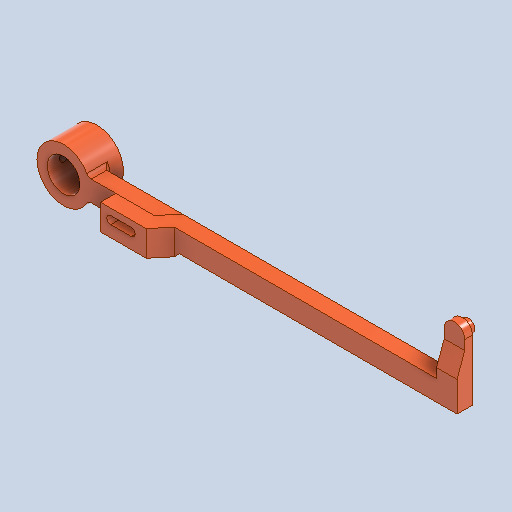
# Autodesk Inventor part: head_lock_2
Saved by Autodesk Inventor 2024 (Build 280153000, 153)
## iProperties
Created: 2021-06-14
Part Number: head_lock_2
Material: Generic
Document SubType Name: Modeling
Designer: dsdan
Density: 1 g/cm^3
Appearance: Smooth - Light Orange
Author: dsdan
Autodesk Inventor part; units mm, degrees
ref_plane "YZ Plane" through (0, 0, 0) normal (1, 0, 0) x (0, 1, 0)
sketch "Sketch1" plane through (0, 0, 0) normal (0, 0, 1) x (1, 0, 0)
  circle A0 centre (7.936401, -24.412437) radius 2.575 construction
  circle A1 centre (7.936401, -24.412437) radius 2.55
  dimension "d70" = 5.1
  constraints: 1 centre point, 1 coincident
  measures "d70" diameter of A1
sketch "Sketch1 outline for Extrusion1" plane through (0, 0, 0) normal (0, 0, 1) x (1, 0, 0)
  circle A0 centre (7.936401, -24.412437) radius 2.55
extrude "Extrusion1" add sketch "Sketch1 outline for Extrusion1" against normal blind 2.4
sketch "Sketch2" plane through (0, 0, 0) normal (0, 0, 1) x (1, 0, 0)
  arc A0 (11.936401, -24.412437) -> (3.936401, -24.412437) centre (7.936401, -24.412437) ccw
  line L0 (11.936401, -24.412437) -> (3.936401, -24.412437) construction
  line L1 (3.936401, -24.412437) -> (3.936401, -40.089664)
  line L2 (11.936401, -48.089664) -> (11.936401, -24.412437)
  line L3 (-141.474726, -48.126865) -> (-141.474726, -40.126865) construction
  line L4 (-131.928915, -40.089664) -> (3.936401, -40.089664)
  arc A1 (-131.928915, -40.089664) -> (-131.928915, -48.089664) centre (-141.474726, -44.089664) ccw
  line L5 (11.936401, -48.089664) -> (-131.928915, -48.089664)
  circle A2 centre (-141.474726, -44.089664) radius 6.35
  line L6 (-118.52781, -40.089664) -> (-118.52781, -48.089664) construction
  circle A3 centre (-141.474726, -44.089664) radius 5.8293
  circle A4 centre (7.936401, -24.412437) radius 2.55
  point P0 (-118.52781, -44.089664)
  point P1 (12.740451, -19.012437)
  dimension "d3" = 8
  dimension "d36" = 12.7
  dimension "d37" = 4
  dimension "d38" = 8
  constraints: 14 end point, 4 point on circle, 3 centre point, 3 coincident, 3 perpendicular, 3 point on line, 2 horizontal, 2 parallel, 2 tangent, 1 concentric, 1 horizontal alignment, 1 midpoint, 1 other
  measures "d3" diameter of A0
  measures "d36" diameter of A2
  measures "d37" radial gap between concentric circles of A1 A2
  measures "d38" distance between parallel lines of L5 L4
sketch "Sketch2 outline for Extrusion2" plane through (0, 0, 0) normal (0, 0, 1) x (1, 0, 0)
  line L0 (11.936401, -48.089664) -> (11.936401, -24.412437)
  line L1 (-131.928915, -48.089664) -> (11.936401, -48.089664)
  arc A0 (11.936401, -24.412437) -> (3.936401, -24.412437) centre (7.936401, -24.412437) ccw
  arc A1 (-131.928915, -40.089664) -> (-131.928915, -48.089664) centre (-141.474726, -44.089664) ccw
  line L2 (3.936401, -24.412437) -> (3.936401, -40.089664)
  line L3 (3.936401, -40.089664) -> (-131.928915, -40.089664)
  circle A2 centre (-141.474726, -44.089664) radius 6.35
extrude "Extrusion2" add sketch "Sketch2 outline for Extrusion2" along normal blind 6
sketch "Sketch3" plane through (3.936401, -40.089664, 0) normal (-1, 0, 0) x (0, 0, 1)
  line L0 (0, 19.677227) -> (6, 19.677227)
  line L1 (3, 19.677227) -> (3, 11.919659)
  line L2 (3, 11.919659) -> (6, 3.677227)
  line L3 (6, 15.677227) -> (6, 19.677227)
  line L4 (6, 15.677227) -> (6, 0)
  point P0 (0, 40.089664)
  point P1 (5, 8)
  dimension "d8" = 160
  dimension "d10" = 16
  constraints: 4 end point, 1 midpoint, 1 perpendicular, 2 other
  measures "d8" angle of L1 L2
  measures "d10" distance of L0.end L2.end
sketch "Sketch3 outline for Extrusion3" plane through (3.936401, -40.089664, 0) normal (-1, 0, 0) x (0, 0, 1)
  line L0 (6, 15.677227) -> (6, 19.677227)
  line L1 (6, 3.677227) -> (6, 15.677227)
  line L2 (3, 11.919659) -> (6, 3.677227)
  line L3 (3, 19.677227) -> (3, 11.919659)
  line L4 (6, 19.677227) -> (3, 19.677227)
extrude "Extrusion3" cut sketch "Sketch3 outline for Extrusion3" against normal through all
ref_plane "Work Plane3" through (-155.900182, -65.296024, -7) normal (0, 0, 1) x (1, 0, 0)
sketch "Sketch8" plane through (-124.033402, -23.677227, 0) normal (0, 0, 1) x (1, 0, 0)
  arc A0 (-7.895513, -16.412437) -> (-7.895513, -24.412437) centre (-17.441324, -20.412437) ccw
  circle A1 centre (-17.441324, -20.412437) radius 6.35
  circle A2 centre (-17.441324, -20.412437) radius 10.35
  point P0 (124.033402, 23.677227)
  point P1 (-7.895513, -24.412437)
  point P2 (-7.895513, -16.412437)
  constraints: 1 centre point, 1 coincident, 1 concentric
sketch "Sketch8 outline for Extrusion8" plane through (-124.033402, -23.677227, 0) normal (0, 0, 1) x (1, 0, 0)
  arc A0 (-7.895513, -24.412437) -> (-7.895513, -16.412437) centre (-17.441324, -20.412437) ccw
  arc A1 (-7.895513, -16.412437) -> (-7.895513, -24.412437) centre (-17.441324, -20.412437) ccw
  circle A2 centre (-17.441324, -20.412437) radius 6.35
extrude "Extrusion8" add sketch "Sketch8 outline for Extrusion8" against normal up to surface (7 mm away)
fillet "Fillet1" radius 2 3 edges at (-131.1247, -44.0897, 0) (-131.9289, -48.0897, 3) (-131.9289, -40.0897, 3)
ref_plane "Work Plane2" through (-151.824726, -44.089664, 0) normal (-1, 0, 0) x (0, 0, 1)
sketch "Sketch9" plane through (-151.824726, -44.089664, 0) normal (-1, 0, 0) x (0, 0, 1)
  circle A0 centre (-0.5, 0) radius 1.8
  line L0 (6, -10.35) -> (6, 10.35) projected
  point P0 (0, 44.089664)
  point P1 (6, 5.02834)
  point P2 (6, -5.02834)
  point P3 (6, 0)
  dimension "d31" = 3.6
  dimension "d41" = 6.5
  constraints: 1 centre point, 1 horizontal alignment, 1 midpoint
  measures "d31" diameter of A0
  measures "d41" distance from line of A0.centre L0
sketch "Sketch9 outline for Extrusion9" plane through (-151.824726, -44.089664, 0) normal (-1, 0, 0) x (0, 0, 1)
  circle A0 centre (-0.5, 0) radius 1.8
extrude "Extrusion9" cut sketch "Sketch9 outline for Extrusion9" against normal up to next
sketch "Sketch10" plane through (11.936401, -48.089664, 0) normal (0, -1, 0) x (1, 0, 0)
  line L0 (-8, 6) -> (-142.616568, 6)
  line L1 (-118, 6) -> (-113, 0)
  line L2 (-8, 0) -> (-141.726842, 0)
  point P0 (-11.936401, 0)
  point P1 (-142.616879, 0)
  point P2 (-143.760295, 0)
  constraints: 2 end point, 2 point on line
surface extrude "ExtrusionSrf1" sketch "Sketch10" against normal through all shown no curves L1
split body "Split1" result two bodies by surface "ExtrusionSrf1" first body at (-134.013926, -50.520758, -1)
sketch "Sketch11" plane through (11.936401, -48.089664, 0) normal (0, -1, 0) x (1, 0, 0)
  line L0 (-8, 6) -> (-118, 6)
  line L1 (-110.18975, 6) -> (-115.18975, 12)
  line L2 (-110.18975, 6) -> (-102.379501, 6) construction
  line L3 (-115.18975, 12) -> (-133, 12)
  line L4 (-133, 12) -> (-133, 6)
  line L5 (-142.616568, 6) -> (-118, 6)
  line L6 (-133, 6) -> (-118, 6)
  line L7 (-118, 6) -> (-113, 0)
  line L8 (-118, 6) -> (-110.18975, 6)
  line L9 (-113, 0) -> (-141.726842, 0)
  line L10 (-113, 0) -> (0, 0)
  point P0 (-11.936401, 0)
  point P1 (-142.616879, 0)
  point P2 (-143.760295, 0)
  dimension "d47" = 6
  dimension "d48" = 6
  dimension "d49" = 15
  dimension "d64" = 6
  constraints: 12 end point, 2 horizontal, 1 collinear, 1 equal length, 1 parallel, 1 perpendicular, 1 point on line
  measures "d47" vertical distance of L1.start L1.end
  measures "d48" distance between parallel lines of L7 L1
  measures "d49" distance from line of L0.end L4
  measures "d64" distance between parallel lines of L10 L0
sketch "Sketch11 outline for Extrusion10" plane through (11.936401, -48.089664, 0) normal (0, -1, 0) x (1, 0, 0)
  line L0 (-115.18975, 12) -> (-133, 12)
  line L1 (-110.18975, 6) -> (-115.18975, 12)
  line L2 (-118, 6) -> (-110.18975, 6)
  line L3 (-133, 6) -> (-118, 6)
  line L4 (-133, 12) -> (-133, 6)
extrude "Extrusion10" add sketch "Sketch11 outline for Extrusion10" against normal up to surface (8 mm away) bodies 3
sketch "Sketch12" plane through (-121.063599, -48.089664, 12) normal (0, 0, 1) x (1, 0, 0)
  line L0 (4, 4) -> (12, 4) construction
  line L1 (4, 2.45) -> (12, 2.45)
  line L2 (12, 5.55) -> (4, 5.55)
  arc A0 (4, 5.55) -> (4, 2.45) centre (4, 4) ccw
  arc A1 (12, 2.45) -> (12, 5.55) centre (12, 4) ccw
  line L3 (0, 0) -> (0, 8)
  line L4 (17.81025, 0) -> (17.81025, 8)
  point P0 (121.063599, 48.089664)
  point P1 (8, 4)
  point P2 (0, 4)
  dimension "d52" = 8
  dimension "d53" = 3.1
  dimension "d54" = 4
  constraints: 8 end point, 4 point on circle, 4 tangent, 2 centre point, 2 midpoint, 1 horizontal, 1 parallel, 1 point on line
  measures "d52" distance of L0.start L0.end
  measures "d53" diameter of A1
  measures "d54" distance from line of L3 L0.start
sketch "Sketch12 outline for Extrusion11" plane through (-121.063599, -48.089664, 12) normal (0, 0, 1) x (1, 0, 0)
  line L0 (4, 2.45) -> (12, 2.45)
  arc A0 (4, 5.55) -> (4, 2.45) centre (4, 4) ccw
  line L1 (12, 5.55) -> (4, 5.55)
  arc A1 (12, 2.45) -> (12, 5.55) centre (12, 4) ccw
extrude "Extrusion11" cut sketch "Sketch12 outline for Extrusion11" against normal through all bodies 3
sketch "Sketch13" plane through (0, 0, 6) normal (0, 0, 1) x (1, 0, 0)
  arc A0 (-109.063599, -45.639664) -> (-109.063599, -42.539664) centre (-109.063599, -44.089664) ccw
  circle A1 centre (-109.063599, -44.089664) radius 2.4
  point P0 (0, 0)
  dimension "d58" = 4.8
  constraints: 1 centre point, 1 coincident
  measures "d58" diameter of A1
sketch "Sketch13 outline for Extrusion12" plane through (0, 0, 6) normal (0, 0, 1) x (1, 0, 0)
  circle A0 centre (-109.063599, -44.089664) radius 2.4
extrude "Extrusion12" cut sketch "Sketch13 outline for Extrusion12" against normal through all bodies 2
chamfer "Chamfer1" distance 0.5 angle 45 1 edges at (-111.4636, -44.0897, 0)
sketch "Sketch14" plane through (11.936401, -48.089664, 0) normal (0, -1, 0) x (1, 0, 0)
  line L0 (-115.18975, 12) -> (-133, 12)
  line L1 (-133, 12) -> (-115.18975, 12)
  line L2 (-133, 0) -> (-133, 12)
  line L3 (-110.18975, 6) -> (-115.18975, 12)
  line L4 (-115.18975, 12) -> (-110.18975, 6)
  line L5 (-110.18975, 0) -> (-110.18975, 6)
  line L6 (-141.726842, 0) -> (-113, 0)
  line L7 (-133, 0) -> (-110.18975, 0)
  point P0 (-11.936401, 0)
  point P1 (-142.616879, 0)
  point P2 (-143.760295, 0)
  constraints: 10 end point, 3 point on line, 2 collinear, 1 horizontal, 1 perpendicular, 1 vertical
sketch "Sketch14 outline for Extrusion13" plane through (11.936401, -48.089664, 0) normal (0, -1, 0) x (1, 0, 0)
  line L0 (-110.18975, 0) -> (-110.18975, 6)
  line L1 (-133, 0) -> (-110.18975, 0)
  line L2 (-133, 12) -> (-133, 0)
  line L3 (-115.18975, 12) -> (-133, 12)
  line L4 (-110.18975, 6) -> (-115.18975, 12)
extrude "Extrusion13" add sketch "Sketch14 outline for Extrusion13" along normal blind 2 bodies 3
chamfer "Chamfer2" distance 2 angle 45 1 edges at (-98.2533, -48.0897, 3)
equation "\"d47\" = d64"
equation "\"d48\" = d47"
body "Srf1"
body "Solid2"
body "Solid3"
